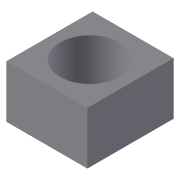
# Autodesk Inventor part: 00_Lens_Iphone_5s
Saved by Autodesk Inventor 2019 (Build 230136000, 136)
## iProperties
Created: 2019-04-26
Part Number: 00_Lens_Iphone_5s
Material: Generic
Document SubType Name: Modeling
Designer: diederichbenedict
Density: 1 g/cm^3
Appearance: Default
Author: diederichbenedict
Autodesk Inventor part; units mm, degrees
ref_plane "YZ Plane" through (0, 0, 0) normal (1, 0, 0) x (0, 1, 0)
ref_plane "XZ Plane" through (0, 0, 0) normal (0, 1, 0) x (-1, 0, 0)
ref_plane "XY Plane" through (0, 0, 0) normal (0, 0, 1) x (1, 0, 0)
sketch "Sketch1" plane through (0, 0, 0) normal (0, 1, 0) x (-1, 0, 0)
  line L0 (3.85, 4.1) -> (-3.85, 4.1)
  line L1 (-3.85, 4.1) -> (-3.85, -4.1)
  line L2 (-3.85, -4.1) -> (3.85, -4.1)
  line L3 (3.85, -4.1) -> (3.85, 4.1)
  line L4 (3.85, 4.1) -> (-3.85, -4.1) construction
  line L5 (-3.85, 4.1) -> (3.85, -4.1) construction
  circle A0 centre (0, 0) radius 2.8472
  dimension "d0" = 7.7
  dimension "d1" = 8.2
  constraints: 12 end point, 2 midpoint, 2 parallel, 1 centre point, 1 coincident, 1 horizontal, 1 perpendicular
  measures "d0" distance of L2.end L1.end
  measures "d1" distance of L1.end L0.end
extrude "Extrusion1" add sketch "Sketch1" along normal blind 5
body "Solid1"
